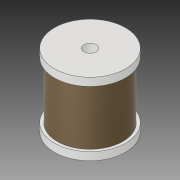
# Autodesk Inventor part: Kupferspule 500g
Saved by Autodesk Inventor 2019.4 (Build 234330000, 330)
## iProperties
Part Number: Kupferspule 500g
Material: PC/ABS-Kunststoff
Document SubType Name: Modeling
Designer: rYan
Density: 0.357273 g/cm^3
Appearance: Glatt - Weiß
Mass: 60.6161 g
Surface Area: 210.879 cm^2
Volume: 169.663 cm^3
Author: rYan
Autodesk Inventor part; units mm, degrees
ref_plane "YZ Plane" through (0, 0, 0) normal (1, 0, 0) x (0, 1, 0)
ref_plane "XZ Plane" through (0, 0, 0) normal (0, 1, 0) x (-1, 0, 0)
ref_plane "XY Plane" through (0, 0, 0) normal (0, 0, 1) x (1, 0, 0)
sketch "Skizze2" plane through (0, 0, 0) normal (0, 1, 0) x (-1, 0, 0)
  line L0 (-5.5, 64) -> (-31.5, 64)
  line L1 (-31.5, 64) -> (-31.5, 57)
  line L2 (-31.5, 57) -> (-29, 57)
  line L3 (-29, 57) -> (-29, 7)
  line L4 (-29, 7) -> (-31.5, 7)
  line L5 (-31.5, 7) -> (-31.5, 0)
  line L6 (-31.5, 0) -> (-5.5, 0)
  line L7 (0, 32) -> (-29, 32) construction
  line L8 (0, 0) -> (0, 64)
  line L9 (-5.5, 64) -> (-5.5, 0)
  point P0 (-5.5, 32)
  dimension "d3" = 7
  dimension "d4" = 64
  dimension "d5" = 11
  dimension "d6" = 63
  dimension "d7" = 58
  constraints: 20 end point, 5 perpendicular, 5 point on line, 2 midpoint, 2 vertical, 1 horizontal, 2 other
  measures "d3" distance of L0.end L1.end
  measures "d4" distance of L0.start L6.end
  measures "d5" diameter of L9 L8
  measures "d6" diameter of L1 L8
  measures "d7" diameter of L3 L8
revolve "Umdrehung1" add sketch "Skizze2" angle 360 about axis through (0, 0, 0) along (0, 0, 1)
